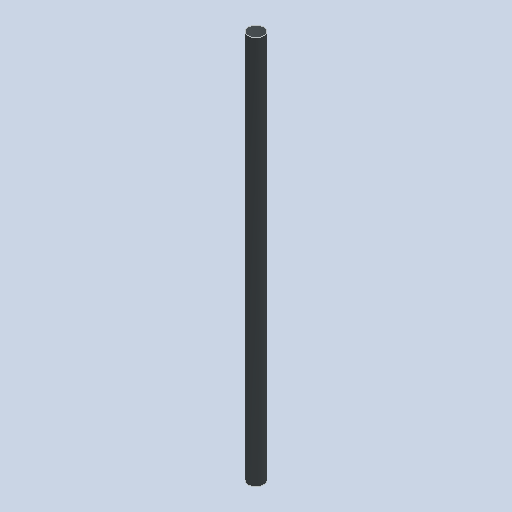
# Autodesk Inventor part: Shaft
Saved by Autodesk Inventor 2022.2 (Build 262287000, 287)
## iProperties
Created: 2022-07-30
Part Number: Shaft
Material: Iron, Cast
Document SubType Name: Modeling
Designer: ABL
Density: 7.15 g/cm^3
Appearance: Iron Gray
Author: ABL
Autodesk Inventor part; units mm, degrees
ref_plane "YZ Plane" through (0, 0, 0) normal (1, 0, 0) x (0, 1, 0)
ref_plane "XZ Plane" through (0, 0, 0) normal (0, 1, 0) x (-1, 0, 0)
ref_plane "XY Plane" through (0, 0, 0) normal (0, 0, 1) x (1, 0, 0)
sketch "Sketch1" plane through (0, 0, 0) normal (0, 1, 0) x (-1, 0, 0)
  circle A0 centre (0, 0) radius 4
  dimension "d0" = 8
  constraints: 1 centre point, 1 coincident
  measures "d0" diameter of A0
extrude "Extrusion1" add sketch "Sketch1" along normal blind 200
equation "\"d0\" = shaftDiameter"
equation "\"d1\" = shaftLength"
equation "\"gap\" = 0.1"
equation "\"airgap\" = 0.4"
equation "\"wallgap\" = 2"
equation "\"driveMagnet_height\" = 5"
equation "\"halbachMagnet_height\" = 3"
equation "\"rotorBandBolt_diameter\" = 2"
equation "\"rotorBandBolt_headDiameter\" = 3.98"
equation "\"rotorBandBolt_headHeight\" = 2"
equation "\"rotorBandHexNut_sideToSide\" = 4"
equation "\"rotorBandHexNut_height\" = 1.2"
equation "\"rotorBandSquareNut_sideLength\" = 4"
equation "\"rotorBandSquareNut_height\" = 1.2"
equation "\"sensorMagnet_diameter\" = 5"
equation "\"sensorMagnet_height\" = 2.66667"
equation "\"rotorRadius\" = 2 * gap + driveMagnet_centerSpacingRadius + driveMagnet_length + wallgap"
equation "\"rotor_mountingLipHeight\" = 0.5 * statorThickness"
equation "\"shaftDiameter\" = 8"
equation "\"flangeBearing_innerDiameter\" = shaftDiameter"
equation "\"flangeBearing_outerDiameter\" = 16"
equation "\"flangeBearing_flangeDiameter\" = 18"
equation "\"flangeBearing_height\" = 5"
equation "\"flangeBearing_flangeHeight\" = 1"
equation "\"statorThickness\" = coilThickness + 2 * wallgap"
equation "\"rotorBandThickness\" = wallgap + rotorBandBolt_headHeight + gap"
equation "\"shaftLength\" = 200"
equation "\"flangeCoupling_collarOuterDiameter\" = 16"
equation "\"flangeCoupling_flangeHoleEdgeToEdge\" = 2.05"
equation "\"flangeCoupling_innerDiameter\" = shaftDiameter"
equation "\"flangeCoupling_flangeHoleDiameter\" = 3.9"
equation "\"flangeCoupling_flangeHeight\" = 3.1"
equation "\"flangeCoupling_flangeDiameter\" = 32"
equation "\"flangeCoupling_height\" = flangeCoupling_collarHeight + flangeCoupling_flangeHeight"
equation "\"flangeCoupling_mountHoleDiameter\" = 3.9"
equation "\"flangeCoupling_mountHoleEdgeToEdge\" = 2.05"
equation "\"statorRadius\" = driveMagnet_length + driveMagnet_centerSpacingRadius + 2 * gap"
equation "\"coilThickness\" = 12"
equation "\"statorMountBolt_diameter\" = 4"
equation "\"statorMountBolt_headDiameter\" = 7"
equation "\"statorMountBolt_headHeight\" = 4"
equation "\"statorMountBolt_shaftLength\" = coilThickness + flangeCoupling_flangeHeight + wallgap"
equation "\"statorMountHexNut_height\" = 4"
equation "\"statorMountHexNut_sideToSide\" = 8"
equation "\"sensorMagnet_ringRadius\" = 0.5 * driveMagnet_centerSpacingRadius + 2 * wallgap"
equation "\"coil_percentCoverage\" = 0.6"
equation "\"statorSpokeDegrees\" = 4deg"
equation "\"coil_bulge\" = 3"
equation "\"statorCoilBolt_shaftLength\" = coilThickness"
equation "\"statorCoilHexNut_height\" = 1.2"
equation "\"statorCoilBolt_headHeight\" = 2"
equation "\"statorCoilBolt_diameter\" = 2"
equation "\"statorCoilBolt_headDiameter\" = 3.98"
equation "\"statorCoilHexNut_sideToSide\" = 4"
equation "\"driveMagnet_centerSpacingRadius\" = 38.96113"
equation "\"driveMagnet_length\" = 60"
equation "\"flangeCoupling_collarHeight\" = 10"
body "Solid1"
